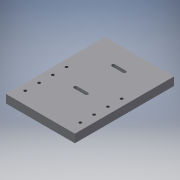
# Autodesk Inventor part: MacroBasePlate_V1
Saved by Autodesk Inventor 2019 (Build 230136000, 136)
## iProperties
Created: 2012-05-23
Part Number: MacroBasePlate_V1
Document SubType Name: Modeling
Designer: Fabian
Density: 1 g/cm^3
Material: Generic
Appearance: Default
Author: Fabian
Autodesk Inventor part; units mm, degrees
ref_plane "YZ Plane" through (0, 0, 0) normal (1, 0, 0) x (0, 1, 0)
ref_plane "XZ Plane" through (0, 0, 0) normal (0, 1, 0) x (-1, 0, 0)
sketch "Sketch1" plane through (0, 0, 0) normal (0, 0, 1) x (1, 0, 0)
  circle A0 centre (5, 95) radius 3 construction
  arc A1 (-53, -30) -> (-47, -30) centre (-50, -30) ccw construction
  line L0 (-53, -30) -> (-53, 30) construction
  arc A2 (-47, 30) -> (-53, 30) centre (-50, 30) ccw construction
  line L1 (-47, 30) -> (-47, -30) construction
  arc A3 (47, -30) -> (53, -30) centre (50, -30) ccw construction
  line L2 (47, -30) -> (47, 30) construction
  arc A4 (53, 30) -> (47, 30) centre (50, 30) ccw construction
  line L3 (53, 30) -> (53, -30) construction
  circle A5 centre (31.5, 31.5) radius 6 construction
  circle A6 centre (-31.5, 31.5) radius 6 construction
  circle A7 centre (-31.5, -31.5) radius 6 construction
  circle A8 centre (31.5, -31.5) radius 6 construction
  line L4 (62.5, 47.5) -> (-62.5, 47.5) construction
  line L5 (-62.5, 47.5) -> (-62.5, -47.5) construction
  line L6 (-62.5, -47.5) -> (62.5, -47.5) construction
  line L7 (62.5, -47.5) -> (62.5, 47.5) construction
  line L8 (62.5, -47.5) -> (-62.5, -47.5)
  line L9 (-62.5, -47.5) -> (-62.5, 132.5)
  line L10 (-62.5, 132.5) -> (62.5, 132.5)
  line L11 (62.5, 132.5) -> (62.5, -47.5)
  point P0 (0, 0)
  dimension "d0" = 180
  dimension "d1" = 125
  constraints: 8 end point, 2 parallel, 1 horizontal, 1 perpendicular
  measures "d0" distance of L8.end L9.end
  measures "d1" distance of L9.end L10.end
ref_plane "Work Plane1" through (-75, -725, 15) normal (0, 0, -1) x (0, 1, 0)
extrude "Extrusion1" add sketch "Sketch1" along normal up to surface (15 mm away)
sketch "Sketch2" plane through (0, 0, 0) normal (0, 0, -1) x (-1, 0, 0)
  line L0 (-62.5, -47.5) -> (62.5, -47.5) projected
  arc A0 (47, -30) -> (53, -30) centre (50, -30) ccw construction
  arc A1 (53, 30) -> (47, 30) centre (50, 30) ccw construction
  line L1 (47, 30) -> (47, -30) construction
  line L2 (53, -30) -> (53, 30) construction
  point P0 (0, 0)
  point P1 (50, -25)
  point P2 (50, 0)
  point P3 (50, 25)
  point P4 (-50, -25)
  point P5 (-50, 0)
  point P6 (-50, 25)
  point P7 (50, 50)
  point P8 (-50, 50)
  dimension "d5" = 55
  dimension "d8" = 25
  dimension "d11" = 100
  constraints: 1 horizontal, 1 vertical, 7 other
  measures "d5" distance of A1.centre point (50, -25)
  measures "d8" distance of point (50, -25) point (50, 0)
  measures "d11" distance of point (50, -25) point (-50, -25)
hole "Hole1" at (-50, -25, 0) at (-50, 0, 0) at (-50, 25, 0) at (50, -25, 0) at (50, 0, 0) at (50, 25, 0) at (-50, 50, 0) at (50, 50, 0) direction (0, 0, 1) diameter 4.917 end through all thread size "M6x1" class "6H" standard "ANSI Metric M Profile"
sketch "Sketch4" plane through (0, 0, 0) normal (0, 0, -1) x (-1, 0, 0)
  circle A0 centre (-5, 95) radius 3 projected
  line L0 (0, -83.5) -> (0, 168.5) projected
  line L1 (-10, 95) -> (10, 95) construction
  line L2 (-10, 92) -> (10, 92)
  line L3 (-10, 98) -> (10, 98)
  arc A1 (10, 92) -> (10, 98) centre (10, 95) ccw
  arc A2 (-10, 98) -> (-10, 92) centre (-10, 95) ccw
  line L4 (-62.5, 47.5) -> (62.5, 47.5) construction
  line L5 (-10, 26.134) -> (10, 26.134) construction
  line L6 (-10, 23.134) -> (10, 23.134)
  line L7 (-10, 29.134) -> (10, 29.134)
  arc A3 (10, 23.134) -> (10, 29.134) centre (10, 26.134) ccw
  arc A4 (-10, 29.134) -> (-10, 23.134) centre (-10, 26.134) ccw
  point P0 (0, 0)
  dimension "d21" = 20
  dimension "d22" = 3
  dimension "d23" = 3
  dimension "d24" = 6
  dimension "d27" = 47.5
  dimension "d30" = 68.866
  constraints: 12 end point, 8 point on circle, 4 centre point, 2 parallel, 2 tangent, 1 perpendicular, 1 vertical, 13 other
  measures "d21" distance of L3.start L3.end
  measures "d22" radius of A2
  measures "d23" radius of A1
  measures "d24" distance between parallel lines of L2 L3
  measures "d27" distance from line of L1.end L4
  measures "d30" distance of L2.start L6.start
extrude "Extrusion2" cut sketch "Sketch4" against normal blind 15
sketch "Sketch5" plane through (0, 0, 0) normal (0, 0, -1) x (-1, 0, 0)
  arc A0 (10, 92) -> (10, 98) centre (10, 95) ccw projected
  line L0 (10, 92) -> (-10, 92) projected
  arc A1 (-10, 98) -> (-10, 92) centre (-10, 95) ccw projected
  line L1 (-10, 98) -> (10, 98) projected
  arc A2 (10, 23.134) -> (10, 29.134) centre (10, 26.134) ccw projected
  line L2 (10, 23.134) -> (-10, 23.134) projected
  arc A3 (-10, 29.134) -> (-10, 23.134) centre (-10, 26.134) ccw projected
  line L3 (-10, 29.134) -> (10, 29.134) projected
  arc A4 (10, 92) -> (10, 98) centre (10, 95) ccw projected
  line L4 (10, 92) -> (-10, 92) projected
  arc A5 (-10, 98) -> (-10, 92) centre (-10, 95) ccw projected
  line L5 (-10, 98) -> (10, 98) projected
  circle A6 centre (-50, 50) radius 2.4585 projected
  circle A7 centre (50, 50) radius 2.4585 projected
  circle A8 centre (-50, 25) radius 2.4585 projected
  circle A9 centre (-50, 0) radius 2.4585 projected
  circle A10 centre (-50, -25) radius 2.4585 projected
  circle A11 centre (50, 25) radius 2.4585 projected
  circle A12 centre (50, 0) radius 2.4585 projected
  circle A13 centre (50, -25) radius 2.4585 projected
  line L6 (-62.5, -47.5) -> (62.5, -47.5) projected
  line L7 (62.5, -47.5) -> (62.5, 132.5) projected
  line L8 (62.5, 132.5) -> (-62.5, 132.5) projected
  line L9 (-62.5, 132.5) -> (-62.5, -47.5) projected
  line L10 (-10, 89) -> (10, 89)
  line L11 (-10, 101) -> (10, 101)
  arc A14 (10, 89) -> (10, 101) centre (10, 95) ccw
  arc A15 (-10, 101) -> (-10, 89) centre (-10, 95) ccw
  line L12 (0, -83.5) -> (0, 168.5) projected
  line L13 (-10, 20.134) -> (10, 20.134)
  line L14 (-10, 32.134) -> (10, 32.134)
  arc A16 (10, 20.134) -> (10, 32.134) centre (10, 26.134) ccw
  arc A17 (-10, 32.134) -> (-10, 20.134) centre (-10, 26.134) ccw
  point P0 (0, 0)
  dimension "d35" = 12
  dimension "d36" = 6
  dimension "d37" = 6
  dimension "d38" = 6
  dimension "d41" = 68.866
  constraints: 8 end point, 8 point on circle, 4 centre point, 2 tangent, 1 parallel, 1 perpendicular, 1 vertical, 10 other
  measures "d35" distance between parallel lines of L11 L10
  measures "d36" distance from line of L10 A1.centre
  measures "d37" radius of A15
  measures "d38" radius of A14
  measures "d41" distance of L10.start L13.start
extrude "Extrusion3" cut sketch "Sketch5" against normal blind 7 contours A0 L1 L12 L11 A14 L10 L0 | L12 L10 A15 L11 L1 A1 L0 | L14 A16 L13 L12 L2 A2 L3 | L12 L3 A3 L2 L13 A17 L14
body "Solid1"
